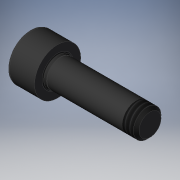
# Autodesk Inventor part: Slotted head cap screw ISO 4762 - M6x20
Saved by Autodesk Inventor 2019 (Build 230136000, 136)
## iProperties
Created: 2022-11-15
Part Number: Slotted head cap screw ISO 4762 - M6x20
Material: Generic
Catalog Web Link: www.cadenas.de
Description: ISO 4762-Hexagon socket head cap screw
Vendor: MISUMI
Document SubType Name: Modeling
Designer: psAdmin
Manufacturer: MISUMI
Mass: 0.942994 g
Surface Area: 7.70071 cm^2
Volume: 0.942994 cm^3
Density: 1 g/cm^3
Appearance: PSOLRGB-175-175-175
Category: PARTsolutions
Company: MISUMI
Title: Slotted head cap screw ISO 4762 - M6x20
Author: Cadenas PARTsolutions
Comments: Hexagon socket head cap screw
PSOL_IDENT_0: {$CADENAS_DATA/23d-libs/misumi/metric/accessories/din_en_iso_4762.prj},221 {VTYP=3D},{NB=Slotted hea
PSOL_IDENT_1: d cap screw ISO 4762 - M6x20},{LINA=Slotted head cap screw ISO 4762 - M6x20},{NN=ISO 4762},{DATE=13.
PSOL_IDENT_2: 07.2021 11:48:40},{GEOMDATE=21.06.2021 06:17:40},{VERSION=},{LINEID=610},{WBVAR=},{WBNUMERIC=}  {NB=
PSOL_IDENT_3: Zylinderschraube ISO 4762 - M6x20},{LINA=Zylinderschraube ISO 4762 - M6x20},{KT=DUMMY},{IDNR=},{D=6.
PSOL_IDENT_4: 000},{D3=4.773},{P=1.000},{L=20.000},{S=5.000},{HM=20.000},{DK=10.000},{DA=6.800},{DS=6.000},{E=5.72
PSOL_IDENT_5: 0},{K=6.000},{R=0.250},{T=3.000},{V=0.600},{DW=9.380},{W=2.300},{LF=0.680},{LG=3.000},{FORM=1.000},{
PSOL_IDENT_6: NENN=M6x20}
NB: Slotted head cap screw ISO 4762 - M6x20
NN: ISO 4762
NT: Hexagon socket head cap screw
NBSYN: Slotted head cap screw ISO 4762 - $NENN.
LINA: Slotted head cap screw ISO 4762 - M6x20
CATALOG: Misumi
ROWDESC: M6x20
D: 6
D3: 4.773
P: 1
L: 20
S: 5
HM: 20
DK: 10
DA: 6.8
DS: 6
E: 5.72
K: 6
R: 0.25
T: 3
V: 0.6
DW: 9.38
W: 2.3
LF: 0.68
LG: 3
FORM: 1
SUPPLIER: MISUMI
ARTICLENO: Slotted head cap screw ISO 4762 - M6x20
BOMINFO: Slotted head cap screw ISO 4762 - M6x20
CREATOR: CADENAS GmbH
Autodesk Inventor part; units mm, degrees
sketch "Skizze_2" plane through (0, 0, 0) normal (0, 0, 1) x (1, 0, 0)
  line L0 (20, 0) -> (-0.8566, 0)
  line L1 (-0.8566, 0) -> (-2.3, 2.5)
  line L2 (-2.3, 2.5) -> (-6, 2.5)
  line L3 (-6, 2.5) -> (-6, 4.4)
  arc A0 (-5.4, 5) -> (-6, 4.4) centre (-5.4, 4.4) ccw
  line L4 (-5.4, 5) -> (0, 5)
  line L5 (0, 5) -> (0, 3.4)
  arc A1 (0, 3.4) -> (0.1677, 3.1639) centre (0.25, 3.4) ccw
  line L6 (0.1677, 3.1639) -> (0.5977, 3.0139)
  arc A2 (0.5977, 3.0139) -> (0.68, 3) centre (0.68, 3.25) ccw
  line L7 (0.68, 3) -> (19.3865, 3)
  line L8 (19.3865, 3) -> (20, 2.3865)
  line L9 (20, 2.3865) -> (20, 0)
  line L10 (20, 0) -> (-0.8566, 0)
  constraints: 22 end point, 6 point on circle, 3 centre point
revolve "Revolution1" add sketch "Skizze_2" angle 360 about axis through (20, 0, 0) along (1, 0, 0)
thread "Thread1" size "M6x1" class "6g" standard "ISO Metric profile" length 2.3865
sketch "Skizze_1" plane through (-2.3, 0, 0) normal (1, 0, 0) x (0, 0, -1)
  line L0 (-2.5, -1.4434) -> (0, -2.8868)
  line L1 (0, -2.8868) -> (2.5, -1.4434)
  line L2 (2.5, -1.4434) -> (2.5, 1.4434)
  line L3 (2.5, 1.4434) -> (0, 2.8868)
  line L4 (0, 2.8868) -> (-2.5, 1.4434)
  line L5 (-2.5, 1.4434) -> (-2.5, -1.4434)
  constraints: 12 end point
extrude "Extrusion1" cut sketch "Skizze_1" against normal blind 6
ref_plane "IP1_XY" through (0, 0, 0) normal (1, 0, 0) x (0, 0, -1)
ref_plane "IP1_YZ" through (0, 0, 0) normal (0, 0, -1) x (0, 1, 0)
ref_plane "IP1_ZX" through (0, 0, 0) normal (0, 1, 0) x (1, 0, 0)
ref_plane "IP2_XY" through (-6, 0, 0) normal (1, 0, 0) x (0, 0, -1)
ref_plane "IP2_YZ" through (-6, 0, 0) normal (0, 0, -1) x (0, 1, 0)
ref_plane "IP2_ZX" through (-6, 0, 0) normal (0, 1, 0) x (1, 0, 0)
ref_plane "IP3_XY" through (20, 0, 0) normal (1, 0, 0) x (0, 0, -1)
ref_plane "IP3_YZ" through (20, 0, 0) normal (0, 0, -1) x (0, 1, 0)
ref_plane "IP3_ZX" through (20, 0, 0) normal (0, 1, 0) x (1, 0, 0)
ref_plane "IP4_XY" through (0, 0, 0) normal (1, 0, 0) x (0, 0, -1)
ref_plane "IP4_YZ" through (0, 0, 0) normal (0, 0, -1) x (0, 1, 0)
ref_plane "IP4_ZX" through (0, 0, 0) normal (0, 1, 0) x (1, 0, 0)
body "Solid1"
